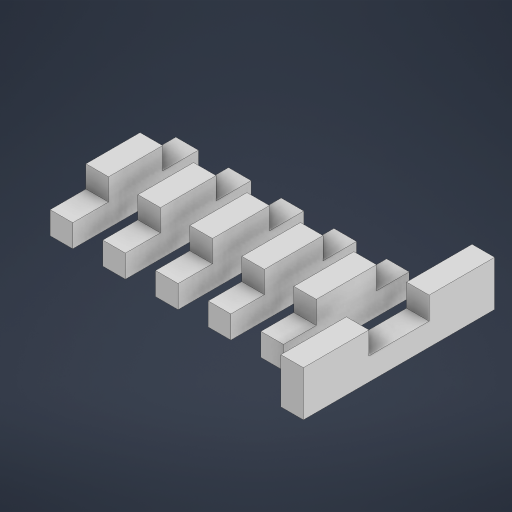
# Autodesk Inventor part: press_fit_test
Saved by Autodesk Inventor 2023 (Build 270158000, 158)
## iProperties
Created: 2022-05-10
Part Number: press_fit_test
Material: Generic
Document SubType Name: Modeling
Designer: Haroon Nawaz
Density: 1 g/cm^3
Appearance: Default
Author: Haroon Nawaz
Autodesk Inventor part; units mm, degrees
ref_plane "YZ Plane" through (0, 0, 0) normal (1, 0, 0) x (0, 1, 0)
ref_plane "XZ Plane" through (0, 0, 0) normal (0, 1, 0) x (-1, 0, 0)
ref_plane "XY Plane" through (0, 0, 0) normal (0, 0, 1) x (1, 0, 0)
sketch "Sketch1" plane through (0, 0, 0) normal (0, 1, 0) x (-1, 0, 0)
  line L0 (0, 0) -> (7.62, 0)
  line L1 (7.62, 0) -> (7.62, -12.7)
  line L2 (7.62, -12.7) -> (0, -12.7)
  line L3 (0, -12.7) -> (0, 0)
  dimension "d0" = 7.62
  dimension "d1" = 12.7
  constraints: 8 end point, 2 parallel, 1 horizontal, 1 perpendicular
  measures "d0" distance of L1.end L2.end
  measures "d1" distance of L0.end L1.end
extrude "Extrusion1" add sketch "Sketch1" along normal blind 3
shell "Shell1" thickness 1.5 removed faces 1 at (-2.54, 3, -4.2333)
sketch "Sketch2" plane through (-6.12, 1.5, -11.2) normal (0, 1, 0) x (1, 0, 0)
  line L0 (0, -9.7) -> (4.62, -9.7) projected
  line L1 (4.62, 0) -> (4.62, -9.7) projected
  line L2 (0, -9.7) -> (4.62, -9.7)
  line L3 (4.62, -9.7) -> (4.62, 0)
  line L4 (4.62, 0) -> (0, 0)
  line L5 (0, 0) -> (0, -9.7)
  point P0 (6.12, -11.2)
  constraints: 8 end point, 2 parallel, 1 horizontal, 1 perpendicular
extrude "Extrusion2" cut sketch "Sketch2" against normal through all
sketch "Sketch3" plane through (0, 0, 0) normal (1, 0, 0) x (0, 0, -1)
  line L0 (0, 3) -> (12.7, 3) projected
  line L1 (4.35, 4.5) -> (8.35, 4.5)
  line L2 (8.35, 4.5) -> (8.35, 1.5)
  line L3 (8.35, 1.5) -> (4.35, 1.5)
  line L4 (4.35, 1.5) -> (4.35, 4.5)
  line L5 (4.35, 4.5) -> (8.35, 1.5) construction
  line L6 (8.35, 4.5) -> (4.35, 1.5) construction
  point P0 (0, 0)
  point P1 (6.35, 3)
  point P2 (8.35, 3)
  point P3 (4.35, 3)
  dimension "d7" = 4
  dimension "d8" = 3
  constraints: 12 end point, 3 midpoint, 2 parallel, 1 horizontal, 1 perpendicular
  measures "d7" distance of L2.end L3.end
  measures "d8" distance of L1.end L2.end
extrude "Extrusion3" cut sketch "Sketch3" against normal through all contours L0 L2 L3 L4
sketch "Sketch4" plane through (-7.62, 0, 0) normal (0, 0, 1) x (1, 0, 0)
  line L0 (2.31, 4.5) -> (5.31, 4.5)
  line L1 (5.31, 4.5) -> (5.31, 1.5)
  line L2 (5.31, 1.5) -> (2.31, 1.5)
  line L3 (2.31, 1.5) -> (2.31, 4.5)
  line L4 (1.5, 3) -> (6.12, 3) projected
  line L5 (2.31, 4.5) -> (5.31, 1.5) construction
  line L6 (5.31, 4.5) -> (2.31, 1.5) construction
  point P0 (7.62, 0)
  point P1 (3.81, 3)
  point P2 (5.31, 3)
  point P3 (2.31, 3)
  dimension "d11" = 3
  dimension "d12" = 3
  constraints: 12 end point, 3 midpoint, 2 parallel, 1 horizontal, 1 perpendicular
  measures "d11" distance of L1.end L2.end
  measures "d12" distance of L0.end L1.end
extrude "Extrusion4" cut sketch "Sketch4" against normal blind 25.4 contours L4 L1 L2 L3
sketch "Sketch6" plane through (-7.62, 0, -12.7) normal (-1, 0, 0) x (0, 0, 1)
  line L0 (4.35, 3) -> (0, 3) projected
  line L1 (0, 3) -> (12.7, 3)
  line L2 (12.7, 3) -> (12.7, 0)
  line L3 (12.7, 0) -> (0, 0)
  line L4 (0, 0) -> (0, 3)
  point P0 (4.35, 3)
  constraints: 8 end point, 2 parallel, 1 horizontal, 1 perpendicular
extrude "Extrusion5" cut sketch "Sketch6" against normal up to surface (6.12 mm away)
ref_plane "Work Plane2" through (-3.5, 0, -12.7) normal (-1, 0, 0) x (0, 0, 1)
sketch "Sketch7" plane through (-3.5, 0, -12.7) normal (-1, 0, 0) x (0, 0, 1)
  line L0 (12.7, 0) -> (0, 0) projected
  line L1 (4.35, 1.5) -> (8.3421, 1.5)
  line L2 (8.3421, 0) -> (4.35, 0)
  line L3 (4.35, 3) -> (0, 3) projected
  line L4 (0, 3) -> (12.7, 3)
  line L5 (12.7, 3) -> (12.7, 0)
  line L6 (12.7, 0) -> (0, 0)
  line L7 (0, 0) -> (0, 3)
  line L8 (4.35, 1.5) -> (4.35, 3)
  line L9 (4.35, 1.5) -> (0, 1.5)
  line L10 (0, 0) -> (0, 3) projected
  line L11 (8.3421, 1.5) -> (12.7, 1.5)
  line L12 (2.175, 1.5) -> (2.175, 0)
  line L13 (10.521, 1.5) -> (10.521, 0)
  line L14 (8.3421, 3) -> (8.3421, 1.5)
  point P0 (4.35, 3)
  constraints: 24 end point, 4 midpoint, 4 point on line, 3 parallel, 3 perpendicular, 2 horizontal, 2 vertical
extrude "Extrusion6" add sketch "Sketch7" along normal blind 1.5 contours L0 L12 L9 L1 L11 L13 | L1 L8 L4 L14
ref_plane "Work Plane3" through (-7, 0, -12.7) normal (-1, 0, 0) x (0, 0, 1)
sketch "Sketch8" plane through (-7, 0, -12.7) normal (-1, 0, 0) x (0, 0, 1)
  line L0 (8.3421, 3) -> (4.35, 3) projected
  line L1 (4.35, 3) -> (4.35, 1.5) projected
  line L2 (4.35, 1.5) -> (2.175, 1.5) projected
  line L3 (2.175, 1.5) -> (2.175, 0) projected
  line L4 (2.175, 0) -> (10.521, 0) projected
  line L5 (10.521, 0) -> (10.521, 1.5) projected
  line L6 (10.521, 1.5) -> (8.3421, 1.5) projected
  line L7 (8.3421, 1.5) -> (8.3421, 3) projected
  line L8 (8.35, 1.5) -> (4.35, 1.5) projected
  line L9 (4.35, 1.5) -> (4.35, 3)
  line L10 (8.3421, 3) -> (4.35, 3)
  line L11 (8.3421, 3) -> (8.35, 1.5)
  line L12 (4.4, 2.95) -> (8.2921, 2.95)
  line L13 (8.2921, 2.95) -> (8.2921, 1.5)
  line L14 (10.421, 1.4) -> (10.421, 0.1)
  line L15 (10.421, 0.1) -> (2.275, 0.1)
  line L16 (2.275, 0.1) -> (2.275, 1.4)
  line L17 (4.4, 1.5) -> (4.4, 2.95)
  line L18 (4.4, 1.5) -> (4.35, 1.5)
  line L19 (8.2921, 1.5) -> (8.35, 1.5)
  point P0 (12.7, 0)
  dimension "d22" = 0.05
  dimension "d46" = 0.05
  dimension "d47" = 0.05
  constraints: 22 end point, 2 collinear, 2 perpendicular, 2 point on line, 2 other
  measures "d22" distance between parallel lines of L0 L12
  measures "d46" distance between parallel lines of L7 L13
  measures "d47" distance between parallel lines of L1 L17
extrude "Extrusion7" add sketch "Sketch8" along normal blind 1.5 contours L6 L5 L4 L3 L2 L8 | L8 L17 L12 L13
pattern_linear "Rectangular Pattern1" count 4 spacing 3.5 along (-1, 0, 0) of "Extrusion7"
thicken "Thicken4" operation cut thickness 0.05 both sides no extend neighbours no toward (0, 0, 1) faces at (-11, 2.4667, -8.3)
thicken "Thicken5" operation cut thickness 0.05 both sides no extend neighbours no toward (0, 0, -1) faces at (-11, 1.9833, -4.4079)
thicken "Thicken6" operation cut thickness 0.1 both sides no extend neighbours no toward (0, 0, -1) faces at (-14.5, 1.9833, -4.4079)
thicken "Thicken7" operation cut thickness 0.1 both sides no extend neighbours no toward (0, 0, 1) faces at (-14.5, 2.4667, -8.3)
thicken "Thicken8" operation cut thickness 0.15 both sides no extend neighbours no toward (0, 0, 1) faces at (-18, 2.4667, -8.3)
thicken "Thicken9" operation cut thickness 0.15 both sides no extend neighbours no toward (0, 0, -1) faces at (-18, 1.9833, -4.4079)
sketch "Sketch11" plane through (-7, 0, -10.525) normal (0, -1, 0) x (1, 0, 0)
  circle A0 centre (-0.6969, 7.2365) radius 0.4
  point P0 (7, 10.525)
  dimension "d58" = 0.8
  constraints: 1 centre point
  measures "d58" diameter of A0
extrude "Extrusion8" cut sketch "Sketch11" against normal blind 1
sketch "Sketch12" plane through (-10.5, 0, -10.525) normal (0, -1, 0) x (1, 0, 0)
  circle A0 centre (-0.7613, 7.3159) radius 0.4
  circle A1 centre (-0.7613, 1.1419) radius 0.4
  point P0 (10.5, 10.525)
  dimension "d54" = 0.8
  dimension "d55" = 0.8
  constraints: 2 centre point
  measures "d54" diameter of A0
  measures "d55" diameter of A1
extrude "Extrusion9" cut sketch "Sketch12" against normal blind 1
sketch "Sketch13" plane through (-14, 0, -10.525) normal (0, -1, 0) x (1, 0, 0)
  point P0 (14, 10.525)
  point P1 (-0.7224, 7.2927)
  point P2 (-0.7224, 4.1371)
  point P3 (-0.7224, 1.0947)
  point P4 (-4.2929, 7.2927)
  point P5 (-4.25, 5.3818)
  point P6 (-4.25, 3.0811)
  point P7 (-4.25, 1.0947)
hole "Hole1" at (-14.7224, 0, -3.2323) at (-14.7224, 0, -6.3879) at (-14.7224, 0, -9.4303) at (-18.2929, 0, -3.2323) at (-18.25, 0, -5.1432) at (-18.25, 0, -7.4439) at (-18.25, 0, -9.4303) direction (0, 1, 0) diameter 0.8 depth 1 tip angle 118
body "Solid1"
